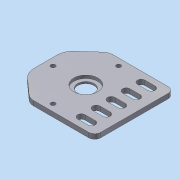
# Autodesk Inventor part: Threaded Rod Plate
Saved by Autodesk Inventor 2013 (Build 170138000, 138)
## iProperties
Created: 2013-12-08
Part Number: Threaded Rod Plate
Material: Aluminum 6061
Document SubType Name: Modeling
Designer: Jon Hollander
Density: 2.71 g/cm^3
Catalog Web Link: www.openbuildspartstore.com
Vendor: OpenBuilds
Mass: 21.0874 g
Surface Area: 63.8132 cm^2
Volume: 7.78134 cm^3
Author: Work
Autodesk Inventor part; units mm, degrees
ref_plane "YZ Plane" through (0, 0, 0) normal (1, 0, 0) x (0, 1, 0)
ref_plane "XZ Plane" through (0, 0, 0) normal (0, 1, 0) x (-1, 0, 0)
ref_plane "XY Plane" through (0, 0, 0) normal (0, 0, 1) x (1, 0, 0)
sketch "Sketch1" plane through (0, 0, 0) normal (0, 0, 1) x (1, 0, 0)
  line L0 (-13.9366, 26.5) -> (29.645, 26.5)
  line L1 (29.645, 26.5) -> (29.645, -26.5)
  line L2 (29.645, -26.5) -> (-13.9366, -26.5)
  line L3 (-29.645, -12.4581) -> (-29.645, 12.4581)
  line L4 (-29.645, 26.5) -> (29.645, -26.5) construction
  line L5 (29.645, 26.5) -> (-29.645, -26.5) construction
  circle A0 centre (-11.1685, 19.25) radius 7.25 construction
  circle A1 centre (-18.965, 7.68) radius 10.68 construction
  line L6 (-29.645, 7.68) -> (29.645, 7.68) construction
  line L7 (29.645, 0) -> (-29.645, 0) construction
  line L8 (29.645, 26.5) -> (-12.105, 26.5) construction
  line L9 (-16.0003, 24.6552) -> (-26.0827, 15.6424) construction
  line L10 (-13.9366, 26.5) -> (-29.645, 12.4581)
  line L11 (-29.645, -12.4581) -> (-13.9366, -26.5)
  line L12 (-13.9366, 26.5) -> (-13.9366, -26.5) construction
  point P0 (0, 0)
  dimension "d3" = 14.5
  dimension "d4" = 21.36
  dimension "d0" = 59.29
  dimension "d2" = 53
  dimension "d6" = 7.68
  dimension "d7" = 41.75
  dimension "d8" = 12.4581
  dimension "d9" = 12.4581
  dimension "d10" = 43.5816
  dimension "d11" = 59.29
  constraints: 26 end point, 4 midpoint, 4 parallel, 4 point on line, 3 perpendicular, 2 horizontal, 1 collinear, 1 vertical, 8 other
  measures "d0" distance of L1.end L5.end
  measures "d2" distance of L0.end L1.end
  measures "d6" distance between parallel lines of L6 L7
  measures "d7" distance of L0.end L8.end
  measures "d8" distance of L7.end L3.end
  measures "d9" distance of L3.start L7.end
  measures "d10" distance between parallel lines of L12 L1
  measures "d11" distance from line of L4.start L1
extrude "Extrusion1" add sketch "Sketch1" along normal mid plane 3.17
sketch "Sketch2" plane through (0, 0, 1.585) normal (0, 0, 1) x (1, 0, 0)
  line L0 (-29.645, 12.4581) -> (-29.645, -12.4581) projected
  line L1 (-13.9366, -26.5) -> (29.645, -26.5) projected
  line L2 (21.025, -17.51) -> (14.215, -17.51)
  line L3 (14.215, -17.51) -> (14.215, -22.51)
  line L4 (14.215, -22.51) -> (21.025, -22.51)
  line L5 (21.025, -22.51) -> (21.025, -17.51)
  line L6 (21.025, -17.51) -> (14.215, -22.51) construction
  line L7 (14.215, -17.51) -> (21.025, -22.51) construction
  arc A0 (14.215, -17.51) -> (14.215, -22.51) centre (14.215, -20.01) ccw
  arc A1 (21.025, -22.51) -> (21.025, -17.51) centre (21.025, -20.01) ccw
  point P0 (0, 0)
  point P1 (17.62, -20.01)
  dimension "d14" = 6.49
  dimension "d15" = 6.81
  dimension "d16" = 5
  dimension "d17" = 11.81
  dimension "d18" = 43.86
  constraints: 12 end point, 4 midpoint, 4 point on circle, 2 centre point, 2 parallel, 1 horizontal, 1 perpendicular
  measures "d14" distance from line of L1 point (17.62, -20.01)
  measures "d15" distance of L3.end L4.end
  measures "d16" distance of L4.end L2.start
  measures "d18" distance from line of L0 A0.centre
extrude "Extrusion2" cut sketch "Sketch2" against normal through all
pattern_linear "Rectangular Pattern1" count 5 spacing 10 along (0, 1, 0) of "Extrusion2"
sketch "Sketch3" plane through (0, 0, 1.585) normal (0, 0, 1) x (1, 0, 0)
  line L0 (-29.645, 12.4581) -> (-29.645, -12.4581) projected
  point P0 (0, 0)
  point P1 (-2.785, 0)
  dimension "d24" = 26.86
  measures "d24" distance from line of L0 point (-2.785, 0)
hole "Hole1" at (-2.785, 0, 1.585) direction (0, 0, -1) diameter 11 end through all counterbore diameter 16.05 counterbore depth 2
sketch "Sketch4" plane through (0, 0, 1.585) normal (0, 0, 1) x (1, 0, 0)
  circle A0 centre (-2.785, 0) radius 8.025 projected
  line L0 (-29.645, 12.4581) -> (-29.645, -12.4581) projected
  point P0 (0, 0)
  point P1 (-2.785, 21.91)
  point P2 (-2.785, -21.91)
  point P3 (-24.685, 0)
  dimension "d34" = 26.86
  dimension "d35" = 43.82
  dimension "d36" = 21.91
  dimension "d37" = 4.96
  dimension "d38" = 21.9
  constraints: 1 horizontal alignment, 1 vertical alignment
  measures "d34" distance from line of L0 point (-2.785, 21.91)
  measures "d35" distance of point (-2.785, -21.91) point (-2.785, 21.91)
  measures "d36" vertical distance of point (-2.785, 21.91) point (-24.685, 0)
  measures "d37" distance from line of L0 point (-24.685, 0)
  measures "d38" distance of A0.centre point (-24.685, 0)
hole "Hole2" at (-2.785, 21.91, 1.585) at (-2.785, -21.91, 1.585) at (-24.685, 0, 1.585) direction (0, 0, -1) diameter 3 end through all
fillet "Fillet1" radius 7.25 1 edges at (-13.9366, -26.5, 0)
fillet "Fillet2" radius 7.25 1 edges at (-13.9366, 26.5, 0)
fillet "Fillet3" radius 10.68 2 edges at (-29.645, 12.4581, 0) (-29.645, -12.4581, 0)
fillet "Fillet4" radius 4 2 edges at (29.645, -26.5, 0) (29.645, 26.5, 0)
equation "\"d9\" = d8"
body "Solid1"
